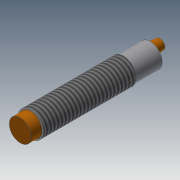
# Autodesk Inventor part: LJ12A3-4-z-BY inductive switch
Saved by Autodesk Inventor 2019 (Build 230136000, 136)
## iProperties
Created: 2019-01-06
Part Number: LJ12A3-4-z-BY inductive switch
Material: Generic
Document SubType Name: Modeling
Designer: LillaHunden
Density: 1 g/cm^3
Appearance: Default
Author: LillaHunden
Autodesk Inventor part; units mm, degrees
ref_plane "YZ Plane" through (0, 0, 0) normal (1, 0, 0) x (0, 1, 0)
ref_plane "XZ Plane" through (0, 0, 0) normal (0, 1, 0) x (-1, 0, 0)
ref_plane "XY Plane" through (0, 0, 0) normal (0, 0, 1) x (1, 0, 0)
sketch "Sketch1" plane through (0, 0, 0) normal (0, 0, 1) x (1, 0, 0)
  circle A0 centre (0, 0) radius 6
  dimension "d0" = 12
  constraints: 1 centre point, 1 coincident
  measures "d0" diameter of A0
extrude "Extrusion1" add sketch "Sketch1" along normal mid plane 43.3
thread "Thread1" size "M12x1.75" class "6g" standard "ISO Metric profile" full length
sketch "Sketch2" plane through (0, 0, 21.65) normal (0, 0, 1) x (1, 0, 0)
  circle A0 centre (0, 0) radius 5.22
  dimension "d5" = 10.44
  constraints: 1 centre point, 1 coincident
  measures "d5" diameter of A0
extrude "Extrusion2" add sketch "Sketch2" along normal blind 5
fillet "Fillet1" radius 0.2 1 edges at (-5.22, 0, 26.65)
fillet "Fillet2" radius 0.2 1 edges at (-5.22, 0, 21.65)
sketch "Sketch3" plane through (0, 0, -21.65) normal (0, 0, -1) x (-1, 0, 0)
  circle A0 centre (0, 0) radius 5.58
  dimension "d10" = 11.16
  constraints: 1 centre point, 1 coincident
  measures "d10" diameter of A0
extrude "Extrusion3" add sketch "Sketch3" along normal blind 12.65
sketch "Sketch4" plane through (0, 0, -34.3) normal (0, 0, -1) x (-1, 0, 0)
  circle A0 centre (0, 2.2194) radius 2.7
  point P0 (0, 0)
  dimension "d13" = 5.4
  constraints: 1 centre point
  measures "d13" diameter of A0
extrude "Extrusion4" add sketch "Sketch4" along normal blind 4.5
draft "FaceDraft1" angle 5 pull direction (0, 0, -1) faces at (-2.6912, 2.0021, -37.3) fixed edges at (2.7, 2.2194, -34.3)
sketch "Sketch5" plane through (0, 0, -34.3) normal (0, 0, -1) x (-1, 0, 0)
  circle A0 centre (0, -3.4527) radius 1.2802
  point P0 (0, 0)
  constraints: 1 centre point
extrude "Extrusion5" add sketch "Sketch5" along normal blind 1.56
fillet "Fillet3" radius 1.2 1 edges at (1.2802, -3.4527, -35.86)
body "Solid1"
